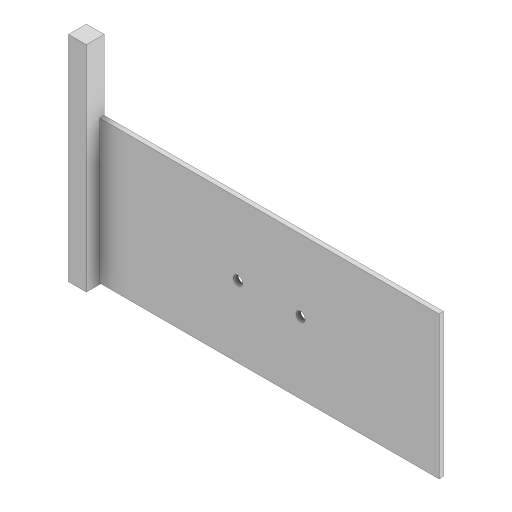
# Autodesk Inventor part: Handle
Saved by Autodesk Inventor 2024.2 (Build 282272000, 272)
## iProperties
Created: 2024-12-02
Part Number: Handle
Material: Generic
Document SubType Name: Modeling
Designer: rhond
Density: 1 g/cm^3
Appearance: Default
Author: rhond
Autodesk Inventor part; units mm, degrees
ref_plane "YZ Plane" through (0, 0, 0) normal (1, 0, 0) x (0, 1, 0)
ref_plane "XZ Plane" through (0, 0, 0) normal (0, 1, 0) x (-1, 0, 0)
ref_plane "XY Plane" through (0, 0, 0) normal (0, 0, 1) x (1, 0, 0)
sketch "Sketch1" plane through (0, 0, 0) normal (0, 0, 1) x (1, 0, 0)
  line L0 (0, 0) -> (241.3, 0)
  line L1 (241.3, 0) -> (241.3, 101.6)
  line L2 (241.3, 101.6) -> (0, 101.6)
  line L3 (0, 101.6) -> (0, 0)
  circle A0 centre (98.425, 50.8) radius 3.175
  circle A1 centre (142.875, 50.8) radius 3.175
  dimension "d0" = 241.3
  dimension "d1" = 101.6
  dimension "d2" = 6.35
  dimension "d3" = 6.35
  dimension "d4" = 44.45
  dimension "d5" = 98.425
  dimension "d6" = 50.8
  constraints: 8 end point, 2 centre point, 2 parallel, 1 horizontal, 1 perpendicular
  measures "d0" distance between parallel lines of L1 L3
  measures "d1" distance of L0.end L1.end
  measures "d2" diameter of A0
  measures "d3" diameter of A1
  measures "d4" distance of A1.centre A0.centre
  measures "d5" distance from line of L3 A0.centre
  measures "d6" distance from line of L2 A1.centre
extrude "Extrusion1" add sketch "Sketch1" along normal blind 3.175
sketch "Sketch2" plane through (0, 0, 0) normal (-1, 0, 0) x (0, 0, 1)
  line L0 (0, -0.8069) -> (12.7, -0.8069)
  line L1 (12.7, -0.8069) -> (12.7, 151.5931)
  line L2 (12.7, 151.5931) -> (0, 151.5931)
  line L3 (0, 151.5931) -> (0, -0.8069)
  line L4 (0, 101.6) -> (0, 0) projected
  dimension "d9" = 12.7
  dimension "d10" = 152.4
  dimension "d11" = 0
  constraints: 8 end point, 2 parallel, 1 horizontal, 1 perpendicular
  measures "d9" distance of L2.end L1.end
  measures "d10" distance of L0.end L1.end
  measures "d11" distance between parallel lines of L3 L4
extrude "Extrusion2" add sketch "Sketch2" along normal blind 12.7
body "Solid1"
